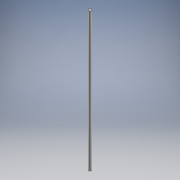
# Autodesk Inventor part: Axel1
Saved by Autodesk Inventor 2017 (Build 210142000, 142)
## iProperties
Created: 2016-10-28
Part Number: Axel1
Material: Generic
Document SubType Name: Modeling
Designer: JJ
Density: 1 g/cm^3
Appearance: Default
Author: JJ
Autodesk Inventor part; units mm, degrees
ref_plane "YZ Plane" through (0, 0, 0) normal (1, 0, 0) x (0, 1, 0)
ref_plane "XZ Plane" through (0, 0, 0) normal (0, 1, 0) x (-1, 0, 0)
ref_plane "XY Plane" through (0, 0, 0) normal (0, 0, 1) x (1, 0, 0)
sketch "Sketch1" plane through (0, 0, 0) normal (0, 0, 1) x (1, 0, 0)
  line L0 (0, -5) -> (0, 5) construction
  line L1 (2.5, -5) -> (2.5, 5)
  line L2 (-2.5, 5) -> (-2.5, -5)
  arc A0 (-2.5, -5) -> (2.5, -5) centre (0, -5) ccw
  arc A1 (2.5, 5) -> (-2.5, 5) centre (0, 5) ccw
  line L3 (-5, 0) -> (5, 0) construction
  line L4 (-5, -2.5) -> (5, -2.5)
  line L5 (5, 2.5) -> (-5, 2.5)
  arc A2 (-5, 2.5) -> (-5, -2.5) centre (-5, 0) ccw
  arc A3 (5, -2.5) -> (5, 2.5) centre (5, 0) ccw
  point P0 (0, 0)
  dimension "d0" = 5
  dimension "d1" = 5
  dimension "d2" = 5
  dimension "d3" = 5
  constraints: 16 end point, 8 point on circle, 8 tangent, 4 centre point, 2 midpoint, 2 parallel, 1 horizontal, 1 vertical
  measures "d0" distance of point (0, 0) L0.end
  measures "d1" diameter of A1
  measures "d2" distance of point (0, 0) L3.end
  measures "d3" diameter of A3
extrude "Extrusion1" add sketch "Sketch1" along normal blind 600
body "Solid1"
